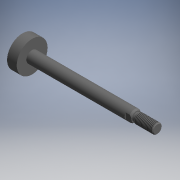
# Autodesk Inventor part: CP96S32-50_ROD
Saved by Autodesk Inventor 2017.3 (Build 213256000, 256)
## iProperties
Part Number: CP96S32-50_ROD
Material: Generic
Catalog Web Link: www.cadenas.de
Description: CP96 ROD-ISO Cylinder:Standard Double Acting,Single/Double Rod
Vendor: SMC
Document SubType Name: Modeling
Designer: partserver
Manufacturer: SMC
Mass: 21.8457 g
Surface Area: 73.5481 cm^2
Volume: 21.8457 cm^3
Density: 1 g/cm^3
Appearance: PSOLRGB-128-128-128
Category: PARTsolutions
Company: SMC
Title: CP96S32-50_ROD
Author: Cadenas PARTsolutions
Comments: ISO Cylinder:Standard Double Acting,Single/Double Rod
PSOL_IDENT_0: {$CADENAS_DATA\23d-libs\smc_jp\actuator\standard_air_cylinder\cp96_c96\cp96\parts\cp96_rod.prj},191
PSOL_IDENT_1: {VTYP=3D},{NB=CP96S32-50_ROD},{LINA=CP96S32-50_ROD},{NN=CP96 ROD},{DATE=05.07.2021 01:48:16},{GEOMDA
PSOL_IDENT_2: TE=30.10.2018 03:42:00},{VERSION=},{LINEID=10},{WBVAR=STROKE,ROD,BOOT},{WBNUMERIC=STROKE}  {NB=CP96S
PSOL_IDENT_3: 32-50_ROD},{LINA=CP96S32-50_ROD},{KT=DUMMY},{BORE=32},{STROKE=50},{ROD=},{BOOT=},{BOOTX='','(-) With
PSOL_IDENT_4: out boot','J','(J) Nylon tarpaulin (one end)','K','(K) Heat resistant tarpaulin (one end)'},{ORDER=C
PSOL_IDENT_5: P96S32-50},{A=22},{B=30},{D=12},{L12=6.0},{KK=M10x1.25},{KKRA=10},{KKRP=1.25},{SW=10},{G=32.0},{L8=9
PSOL_IDENT_6: 4},{H=48},{RR=1},{LD1=10},{A1=2.00},{LD2=8.4},{HB=75},{HB1=75.000},{HB2=88.000},{HB3=100.000},{HB4=1
PSOL_IDENT_7: 13.000},{HB5=138.000},{HB6=163.000},{HB7=188.000},{HB8=213.000},{HB9=238.000},{HB10=263.000},{HB11=2
PSOL_IDENT_8: 88.000},{HB12=313.000}
NB: CP96S32-50_ROD
NN: CP96 ROD
NT: ISO Cylinder:Standard Double Acting,Single/Double Rod
NBSYN: $ORDER._ROD
LINA: CP96S32-50_ROD
CATALOG: SMC (JP
BORE: 32
STROKE: 50
ROD: (-) Single rod
BOOT: (-) Without boot
A: 22
B: 30
D: 12
L12: 6
KK: M10x1.25
SW: 10
G: 32
L8: 94
H: 48
RR: 1
LD1: 10
HB1: 75
HB2: 88
HB3: 100
HB4: 113
HB5: 138
HB6: 163
HB7: 188
HB8: 213
HB9: 238
HB10: 263
HB11: 288
HB12: 313
SUPPLIER: SMC
ARTICLENO: CP96S32-50_ROD
BOMINFO: CP96S32-50_ROD
CREATOR: CADENAS GmbH
Autodesk Inventor part; units mm, degrees
sketch "Sketch_1" plane through (0, 0, 0) normal (0, 0, 1) x (1, 0, 0)
  line L0 (92, 0) -> (-48, 0)
  line L1 (-48, 0) -> (-48, 4.233)
  line L2 (-48, 4.233) -> (-47.233, 5)
  line L3 (-47.233, 5) -> (-28.767, 5)
  line L4 (-28.767, 5) -> (-28, 4.233)
  line L5 (-28, 4.233) -> (-28, 4.2)
  line L6 (-28, 4.2) -> (-26, 4.2)
  line L7 (-26, 4.2) -> (-26, 5)
  line L8 (-26, 5) -> (-24.2679, 6)
  line L9 (-24.2679, 6) -> (82, 6)
  line L10 (82, 6) -> (82, 16)
  line L11 (82, 16) -> (92, 16)
  line L12 (92, 16) -> (92, 0)
  line L13 (92, 0) -> (-48, 0)
  constraints: 28 end point
revolve "Revolution1" add sketch "Sketch_1" angle 360 about axis through (92, 0, 0) along (1, 0, 0)
thread "Thread1" size "M10x1.25" class "6g" standard "ISO Metric profile" full length
sketch "Sketch_4" plane through (-26, 0, 0) normal (1, 0, 0) x (0, 0, -1)
  line L0 (-13, -10) -> (13, -10)
  line L1 (13, -10) -> (13, 10)
  line L2 (13, 10) -> (-13, 10)
  line L3 (-13, 10) -> (-13, -10)
  line L4 (-8, 5) -> (-8, -5)
  line L5 (-8, -5) -> (8, -5)
  line L6 (8, -5) -> (8, 5)
  line L7 (8, 5) -> (-8, 5)
  constraints: 16 end point
extrude "Extrusion1" cut sketch "Sketch_4" along normal blind 6
ref_plane "A4_XY" through (220, 0, 0) normal (0, 1, 0) x (1, 0, 0)
ref_plane "A4_YZ" through (220, 0, 0) normal (1, 0, 0) x (0, 0, -1)
ref_plane "A4_ZX" through (220, 0, 0) normal (0, 0, -1) x (0, 1, 0)
ref_plane "ROD_BODY_XY" through (0, 0, 0) normal (1, 0, 0) x (0, 0, -1)
ref_plane "ROD_BODY_YZ" through (0, 0, 0) normal (0, 0, -1) x (0, 1, 0)
ref_plane "ROD_BODY_ZX" through (0, 0, 0) normal (0, 1, 0) x (1, 0, 0)
ref_plane "ROD_NUT_XY" through (-48, 0, 0) normal (-1, 0, 0) x (0, 0, -1)
ref_plane "ROD_NUT_YZ" through (-48, 0, 0) normal (0, 0, -1) x (0, -1, 0)
ref_plane "ROD_NUT_ZX" through (-48, 0, 0) normal (0, -1, 0) x (-1, 0, 0)
body "Solid1"
